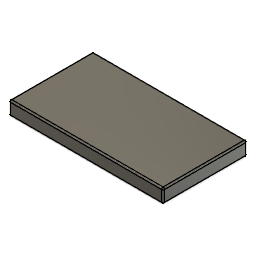
WirelessQAZ_CASE_MAIN v22 (Autodesk Fusion 360 archive; units mm, degrees)
design "Battery Mockup"
Autodesk Fusion 360 part; units mm, degrees
sketch "Sketch1" plane through (0, 0, 0) normal (0, 1, 0) x (1, 0, 0)
  line L0 (27.5, 15) -> (-27.5, 15)
  line L1 (-27.5, 15) -> (-27.5, -15)
  line L2 (-27.5, -15) -> (27.5, -15)
  line L3 (27.5, -15) -> (27.5, 15)
  line L4 (27.5, 15) -> (-27.5, -15) construction
  line L5 (-27.5, 15) -> (27.5, -15) construction
  dimension "d1" = 55
  dimension "d2" = 30
  constraint horizontal L0
  constraint perpendicular L0 L1
  constraint parallel L0 L2
  constraint parallel L1 L3
  constraint coincident L4 origin
  constraint coincident L5 origin
  measures "d1" distance of L1.end L2.end
  measures "d2" distance of L0.end L1.end
extrude "Extrude1" add sketch "Sketch1" along normal blind 5
fillet "Fillet1" radius 0.5 12 edges at (0, 5, 15) (-27.5, 5, 0) (0, 5, -15) (27.5, 5, 0) (27.5, 2.5, -15) (27.5, 2.5, 15) (-27.5, 2.5, 15) (-27.5, 2.5, -15) (0, 0, 15) (-27.5, 0, 0) (0, 0, -15) (27.5, 0, 0)
